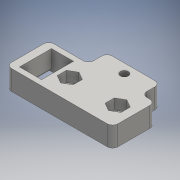
# Autodesk Inventor part: optical endstop base
Saved by Autodesk Inventor 2016 SP1 (Build 200210100, 210)
## iProperties
Created: 2016-04-16
Part Number: optical endstop base
Material: Generic
Document SubType Name: Modeling
Designer: ubik
Density: 1 g/cm^3
Appearance: Default
Author: ubik
Autodesk Inventor part; units mm, degrees
ref_plane "YZ Plane" through (0, 0, 0) normal (1, 0, 0) x (0, 1, 0)
ref_plane "XZ Plane" through (0, 0, 0) normal (0, 1, 0) x (-1, 0, 0)
ref_plane "XY Plane" through (0, 0, 0) normal (0, 0, 1) x (1, 0, 0)
sketch "Sketch1" plane through (0, 0, 0) normal (0, 0, 1) x (1, 0, 0)
  line L0 (-10.2, 5) -> (-10.2, -5) projected
  line L1 (-10.2, -5) -> (16.5, -5) projected
  line L2 (16.5, -5) -> (16.5, 5) projected
  line L3 (16.5, 5) -> (-10.2, 5) projected
  circle A0 centre (13.4, 0) radius 1.5 projected
  circle A1 centre (-4.6, 0) radius 1.5 projected
  line L4 (-16.5, 5) -> (-16.5, -5) projected
  line L5 (-20.5, 8) -> (19.5, 8)
  line L6 (19.5, 8) -> (19.5, -8)
  line L7 (19.5, -8) -> (-20.5, -8)
  line L8 (-20.5, -8) -> (-20.5, 8)
  line L9 (-9.2, 8) -> (-9.2, -8)
  line L10 (-17.5, 8) -> (-17.5, -8)
  line L11 (-17.5, 6) -> (-9.2, 6)
  line L12 (-17.5, -6) -> (-9.2, -6)
  point P0 (0, 0)
  dimension "d0" = 3
  dimension "d1" = 3
  dimension "d2" = 3
  dimension "d3" = 4
  dimension "d4" = 1
  dimension "d5" = 1
  dimension "d6" = 1
  dimension "d7" = 1
  constraints: 16 end point, 8 point on line, 5 perpendicular, 2 parallel, 1 horizontal
  measures "d0" distance between parallel lines of L3 L5
  measures "d1" distance between parallel lines of L7 L1
  measures "d2" distance between parallel lines of L2 L6
  measures "d3" distance between parallel lines of L4 L8
  measures "d4" distance between parallel lines of L9 L0
  measures "d5" distance between parallel lines of L4 L10
  measures "d6" distance between parallel lines of L3 L11
  measures "d7" distance between parallel lines of L1 L12
extrude "Extrusion1" add sketch "Sketch1" along normal blind 7.5 contours L9 L5 L6 L7 L1 L2 L3 | L3 L2 L1 L9 | L11 L10 L5 L9 | L9 L7 L10 L12 | L10 L7 L8 L5
sketch "Sketch2" plane through (0, 0, 7.5) normal (0, 0, 1) x (1, 0, 0)
  circle A0 centre (-4.6, 0) radius 1.5 projected
  circle A1 centre (13.4, 0) radius 1.5 projected
  line L0 (-1.6, -1.7321) -> (-4.6, -3.4641)
  line L1 (-4.6, -3.4641) -> (-7.6, -1.7321)
  line L2 (-7.6, -1.7321) -> (-7.6, 1.7321)
  line L3 (-7.6, 1.7321) -> (-4.6, 3.4641)
  line L4 (-4.6, 3.4641) -> (-1.6, 1.7321)
  line L5 (-1.6, 1.7321) -> (-1.6, -1.7321)
  circle A2 centre (13.4, 0) radius 1.5 projected
  line L6 (10.4, 1.7321) -> (13.4, 3.4641)
  line L7 (13.4, 3.4641) -> (16.4, 1.7321)
  line L8 (16.4, 1.7321) -> (16.4, -1.7321)
  line L9 (16.4, -1.7321) -> (13.4, -3.4641)
  line L10 (13.4, -3.4641) -> (10.4, -1.7321)
  line L11 (10.4, -1.7321) -> (10.4, 1.7321)
  point P0 (0, 0)
  dimension "d10" = 6
  dimension "d11" = 6
  constraints: 24 end point, 2 coincident, 26 other
  measures "d10" distance between parallel lines of L5 L2
  measures "d11" distance between parallel lines of L8 L11
extrude "Extrusion2" cut sketch "Sketch2" against normal blind 4
sketch "Sketch3" plane through (-20.5, 8, 0) normal (0, 1, 0) x (1, 0, 0)
  line L0 (40, 0) -> (0, 0) projected
  line L1 (0, -7.5) -> (40, -7.5) projected
  line L2 (34.9, 0) -> (14.9, 0)
  line L3 (14.9, 0) -> (14.9, -7.5)
  line L4 (14.9, -7.5) -> (34.9, -7.5)
  line L5 (34.9, -7.5) -> (34.9, 0)
  line L6 (13.1, 5) -> (13.1, 2) projected
  line L7 (13.1, 2) -> (36.7, 2) projected
  line L8 (36.7, 2) -> (36.7, 5) projected
  line L9 (36.7, 5) -> (30.7, 5) projected
  line L10 (30.7, 5) -> (30.7, 13) projected
  line L11 (30.7, 13) -> (26.3, 13) projected
  line L12 (26.3, 13) -> (26.3, 5) projected
  line L13 (26.3, 5) -> (23.5, 5) projected
  line L14 (23.5, 5) -> (23.5, 13) projected
  line L15 (23.5, 13) -> (19.1, 13) projected
  line L16 (19.1, 13) -> (19.1, 5) projected
  line L17 (19.1, 5) -> (13.1, 5) projected
  line L18 (24.9, 15.273) -> (24.9, -16.6011) construction
  point P0 (20.5, 0)
  dimension "d14" = 20
  dimension "d15" = 2.8
  dimension "d16" = 1.4
  dimension "d17" = 10
  constraints: 10 end point, 2 parallel, 2 point on line, 1 horizontal, 1 perpendicular, 1 vertical
  measures "d14" distance between parallel lines of L3 L5
  measures "d15" distance between parallel lines of L14 L12
  measures "d16" distance between parallel lines of L18 L12
  measures "d17" distance between parallel lines of L18 L5
extrude "Extrusion3" add sketch "Sketch3" along normal blind 7 contours L5 L1 L3 L0
sketch "Sketch4" plane through (0, 0, 0) normal (0, 0, -1) x (-1, 0, 0)
  circle A0 centre (-4.4, 11.5) radius 1.5
  line L0 (-19.5, 8) -> (-14.4, 8) projected
  line L1 (-19.5, -8) -> (-19.5, 8) projected
  line L2 (20.5, -8) -> (-19.5, -8) projected
  line L3 (20.5, 8) -> (20.5, -8) projected
  line L4 (5.6, 8) -> (20.5, 8) projected
  line L5 (5.6, 8) -> (5.6, 15) projected
  line L6 (-14.4, 15) -> (5.6, 15) projected
  line L7 (-14.4, 8) -> (-14.4, 15) projected
  circle A1 centre (4.6, 0) radius 1.5 projected
  circle A2 centre (-13.4, 0) radius 1.5 projected
  line L8 (17.5, -6) -> (17.5, 6) projected
  line L9 (9.2, -6) -> (17.5, -6) projected
  line L10 (9.2, 6) -> (9.2, -6) projected
  line L11 (17.5, 6) -> (9.2, 6) projected
  point P0 (0, 0)
  dimension "d20" = 3
  dimension "d21" = 20
  dimension "d22" = 7
  dimension "d23" = 3.5
  dimension "d24" = 10
  constraints: 1 centre point
  measures "d20" diameter of A0
  measures "d21" distance of L6.start L5.end
  measures "d22" distance of L0.end L6.start
  measures "d23" distance from line of L6 A0.centre
  measures "d24" distance from line of L5 A0.centre
extrude "Extrusion4" cut sketch "Sketch4" against normal through all contours A0
fillet "Fillet1" radius 2 8 edges at (-5.6, 15, 3.75) (-5.6, 8, 3.75) (-20.5, 8, 3.75) (-20.5, -8, 3.75) (19.5, -8, 3.75) (19.5, 8, 3.75) (14.4, 8, 3.75) (14.4, 15, 3.75)
sketch "Sketch5" plane through (0, 0, 0) normal (0, 0, -1) x (-1, 0, 0)
  line L0 (18.3, -6) -> (-18.3, -6)
  line L1 (-18.3, -6) -> (-18.3, 6)
  line L2 (-18.3, 6) -> (18.3, 6)
  line L3 (18.3, 6) -> (18.3, -6)
  point P0 (0, 0)
  dimension "d28" = 12
  dimension "d29" = 36.6
  dimension "d30" = 18.3
  dimension "d31" = 6
  constraints: 8 end point, 2 parallel, 1 horizontal, 1 perpendicular
  measures "d28" distance of L2.end L0.start
  measures "d29" distance of L0.start L0.end
  measures "d30" distance from line of point (0, 0) L3
  measures "d31" distance from line of point (0, 0) L0
extrude "Extrusion5" cut sketch "Sketch5" against normal blind 1
equation "\"d1\" = d0"
equation "\"d2\" = d0"
equation "\"d11\" = d10"
equation "\"d16\" = 0.5 * d15"
equation "\"d17\" = 0.5 * d14"
equation "\"d23\" = 0.5 * d22"
equation "\"d24\" = 0.5 * d21"
equation "\"d30\" = 0.5 * d29"
equation "\"d31\" = 0.5 * d28"
body "Solid1"
